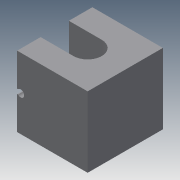
# Autodesk Inventor part: uchyty_robot
Saved by Autodesk Inventor 2013 (Build 170138000, 138)
## iProperties
Created: 2013-05-14
Part Number: uchyty_robot
Material: Generic
Document SubType Name: Modeling
Designer: idle-rug
Density: 1 g/cm^3
Author: idle-rug
Autodesk Inventor part; units mm, degrees
ref_plane "YZ Plane" through (0, 0, 0) normal (1, 0, 0) x (0, 1, 0)
ref_plane "XZ Plane" through (0, 0, 0) normal (0, 1, 0) x (-1, 0, 0)
ref_plane "XY Plane" through (0, 0, 0) normal (0, 0, 1) x (1, 0, 0)
sketch "Sketch1" plane through (0, 0, 0) normal (0, 1, 0) x (-1, 0, 0)
  line L0 (15, 10) -> (-15, 10)
  line L1 (-15, 10) -> (-15, -10)
  line L2 (-15, -10) -> (15, -10)
  line L3 (15, -10) -> (15, 10)
  line L4 (15, 10) -> (-15, -10) construction
  line L5 (-15, 10) -> (15, -10) construction
  point P0 (0, 0)
  dimension "d0" = 30
  dimension "d1" = 20
  constraints: 12 end point, 2 midpoint, 2 parallel, 1 horizontal, 1 perpendicular
  measures "d0" distance of L2.end L1.end
  measures "d1" distance of L1.end L0.end
extrude "Extrusion1" add sketch "Sketch1" along normal blind 10
sketch "Sketch2" plane through (0, 10, 0) normal (0, 1, 0) x (1, 0, 0)
  line L0 (-15, 10) -> (-15, -10) projected
  line L1 (-15, 0) -> (-12, 0)
  circle A0 centre (-13.5, 0) radius 1.5
  point P0 (0, 0)
  dimension "d4" = 3
  constraints: 2 end point, 2 midpoint, 1 centre point, 1 perpendicular, 1 tangent
  measures "d4" distance of L1.start L1.end
extrude "Extrusion2" cut sketch "Sketch2" against normal blind 10
sketch "Sketch3" plane through (0, 10, 0) normal (0, 1, 0) x (1, 0, 0)
  line L0 (-15, 10) -> (-15, 0) projected
  circle A0 centre (-13.5, 0) radius 1.5 projected
  line L1 (-15, 0) -> (-15, -10) projected
  line L2 (-15, 0) -> (-15, 1)
  line L3 (-15, 1) -> (-14.618, 1)
  line L4 (-15, 0) -> (-15, -1)
  line L5 (-15, -1) -> (-14.618, -1)
  point P0 (0, 0)
  dimension "d7" = 1
  dimension "d8" = 1
  constraints: 8 end point, 2 perpendicular, 2 point on circle, 2 point on line
  measures "d7" distance of L0.end L2.end
  measures "d8" distance of L0.end L4.end
extrude "Extrusion3" add sketch "Sketch3" against normal blind 10 contours L3 A0 L0 | A0 L5 L1
sketch "Sketch4" plane through (0, 10, 0) normal (0, 1, 0) x (1, 0, 0)
  circle A0 centre (-13.5, 0) radius 1.5 projected
  line L0 (-15.382, 1) -> (-14.618, 1)
  line L1 (-14.618, 1) -> (-14.618, -1)
  line L2 (-14.618, -1) -> (-15.382, -1)
  line L3 (-15.382, -1) -> (-15.382, 1)
  line L4 (-15.382, 1) -> (-14.618, -1) construction
  line L5 (-14.618, 1) -> (-15.382, -1) construction
  point P0 (0, 0)
  dimension "d11" = 2
  constraints: 12 end point, 2 parallel, 1 horizontal, 1 perpendicular, 2 other
  measures "d11" distance of L0.end L1.end
extrude "Extrusion4" cut sketch "Sketch4" against normal blind 10 contours L1 A0 | A0 L2 L3 L0 picked at (-14.7453, 0)
sketch "Sketch5" plane through (0, 0, 0) normal (0, -1, 0) x (1, 0, 0)
  line L0 (-15, 10) -> (15, 10) projected
  line L1 (15, -10) -> (5, -10)
  line L2 (5, -10) -> (5, 10)
  line L3 (5, 10) -> (15, 10)
  line L4 (15, 10) -> (15, -10)
  point P0 (0, 0)
  dimension "d14" = 10
  constraints: 8 end point, 2 parallel, 1 horizontal, 1 perpendicular, 1 point on line
  measures "d14" distance of L2.end L3.end
extrude "Extrusion5" add sketch "Sketch5" along normal blind 12
sketch "Sketch6" plane through (15, 10, 10) normal (1, 0, 0) x (0, 0, -1)
  line L0 (0, -22) -> (20, -22)
  line L1 (20, -22) -> (20, -32)
  line L2 (20, -32) -> (0, -32)
  line L3 (0, -32) -> (0, -22)
  point P0 (10, -10)
  dimension "d17" = 10
  constraints: 8 end point, 2 parallel, 1 horizontal, 1 perpendicular
  measures "d17" distance of L0.end L1.end
extrude "Extrusion6" add sketch "Sketch6" against normal blind 30
sketch "Sketch7" plane through (15, -22, -10) normal (0, -1, 0) x (1, 0, 0)
  circle A0 centre (-28.5, 10) radius 1.5
  point P0 (-15, 10)
  constraints: 1 centre point
extrude "Extrusion7" cut sketch "Sketch7" against normal blind 10
sketch "Sketch8" plane through (15, -22, -10) normal (0, -1, 0) x (1, 0, 0)
  circle A0 centre (-28.5, 10) radius 1.5 projected
  line L0 (-30.382, 11) -> (-29.618, 11)
  line L1 (-29.618, 11) -> (-29.618, 9)
  line L2 (-29.618, 9) -> (-30.382, 9)
  line L3 (-30.382, 9) -> (-30.382, 11)
  line L4 (-30.382, 11) -> (-29.618, 9) construction
  line L5 (-29.618, 11) -> (-30.382, 9) construction
  point P0 (-15, 10)
  dimension "d23" = 2
  constraints: 12 end point, 2 parallel, 1 horizontal, 1 perpendicular, 2 other
  measures "d23" distance of L0.end L1.end
extrude "Extrusion8" cut sketch "Sketch8" against normal blind 10 contours L1 A0 | A0 L2 L3 L0 picked at (-29.7453, 10)
fillet "Fillet1" radius 6 2 edges at (5, 0, 0) (5, -12, 0)
sketch "Sketch9" plane through (15, 10, -10) normal (0, 0, -1) x (-1, 0, 0)
  line L0 (16, -10) -> (30, -10) projected
  line L1 (30, -10) -> (30, 0) projected
  line L2 (0, 0) -> (30, 0) projected
  line L3 (0, -32) -> (0, 0) projected
  line L4 (0, -32) -> (30, -32) projected
  line L5 (30, -22) -> (30, -32) projected
  line L6 (16, -22) -> (30, -22) projected
  arc A0 (16, -10) -> (16, -22) centre (16, -16) ccw projected
  point P0 (15, -10)
extrude "Extrusion9" add sketch "Sketch9" along normal blind 5
sketch "Sketch10" plane through (-15, 10, 10) normal (0, 0, 1) x (1, 0, 0)
  line L0 (0, -10) -> (14, -10) projected
  arc A0 (14, -22) -> (14, -10) centre (14, -16) ccw projected
  line L1 (14, -22) -> (0, -22) projected
  line L2 (0, -32) -> (0, -22) projected
  line L3 (30, -32) -> (0, -32) projected
  line L4 (30, -32) -> (30, 0) projected
  line L5 (0, 0) -> (30, 0) projected
  line L6 (0, -10) -> (0, 0) projected
  point P0 (15, -10)
extrude "Extrusion10" add sketch "Sketch10" along normal blind 5
sketch "Sketch12" plane through (-15, 10, 10) normal (-1, 0, 0) x (0, 0, 1)
  circle A0 centre (-2, -27) radius 1.5
  point P0 (-10, -10)
  dimension "d31" = 3
  constraints: 1 centre point
  measures "d31" diameter of A0
sketch "Sketch13" plane through (-15, 10, 10) normal (-1, 0, 0) x (0, 0, 1)
  circle A0 centre (-18, -27) radius 1.5
  point P0 (-10, -10)
  dimension "d32" = 3
  constraints: 1 centre point
  measures "d32" diameter of A0
sketch "Sketch14" plane through (-15, 0, -1) normal (-1, 0, 0) x (0, 0, 1)
  circle A0 centre (-7, 5) radius 1.5
  point P0 (1, 0)
  dimension "d33" = 3
  constraints: 1 centre point
  measures "d33" diameter of A0
sketch "Sketch15" plane through (-15, 0, 1) normal (-1, 0, 0) x (0, 0, 1)
  circle A0 centre (7, 5) radius 1.5
  point P0 (-1, 0)
  dimension "d34" = 3
  constraints: 1 centre point
  measures "d34" diameter of A0
extrude "Extrusion11" cut sketch "Sketch14" against normal blind 5
extrude "Extrusion12" cut sketch "Sketch15" against normal blind 5
extrude "Extrusion13" cut sketch "Sketch13" against normal blind 5
extrude "Extrusion14" cut sketch "Sketch12" against normal blind 5
sketch "Sketch17" plane through (-15, 10, 10) normal (-1, 0, 0) x (0, 0, 1)
  circle A0 centre (-2, -27) radius 1.5 projected
  point P0 (-10, -10)
sketch "Sketch18" plane through (-15, 10, 10) normal (-1, 0, 0) x (0, 0, 1)
  circle A0 centre (-18, -27) radius 1.5 projected
  point P0 (-10, -10)
sketch "Sketch19" plane through (-15, 0, -1) normal (-1, 0, 0) x (0, 0, 1)
  circle A0 centre (-7, 5) radius 1.5 projected
  point P0 (1, 0)
sketch "Sketch20" plane through (-15, 0, 1) normal (-1, 0, 0) x (0, 0, 1)
  circle A0 centre (7, 5) radius 1.5 projected
  point P0 (-1, 0)
extrude "Extrusion15" add sketch "Sketch18" against normal blind 5
extrude "Extrusion16" add sketch "Sketch17" against normal blind 5
extrude "Extrusion17" add sketch "Sketch19" against normal blind 5
extrude "Extrusion18" add sketch "Sketch20" against normal blind 5
sketch "Sketch21" plane through (-15, 10, 10) normal (-1, 0, 0) x (0, 0, 1)
  line L0 (-9, -22) -> (5, -22) projected
  line L1 (-2, -22) -> (-2, -26)
  circle A0 centre (-2, -26) radius 1.5
  point P0 (-10, -10)
  dimension "d51" = 4
  dimension "d52" = 3
  constraints: 2 end point, 1 centre point, 1 coincident, 1 midpoint
  measures "d51" distance of L1.start L1.end
  measures "d52" diameter of A0
sketch "Sketch22" plane through (-15, 10, 10) normal (-1, 0, 0) x (0, 0, 1)
  line L0 (-11, -22) -> (-25, -22) projected
  line L1 (-18, -22) -> (-18, -26)
  circle A0 centre (-18, -26) radius 1.5
  point P0 (-10, -10)
  dimension "d53" = 4
  dimension "d54" = 3
  constraints: 2 end point, 1 centre point, 1 coincident, 1 midpoint
  measures "d53" distance of L1.start L1.end
  measures "d54" diameter of A0
sketch "Sketch23" plane through (-15, 0, -1) normal (-1, 0, 0) x (0, 0, 1)
  line L0 (0, 0) -> (-14, 0) projected
  line L1 (-7, 0) -> (-7, 4)
  circle A0 centre (-7, 4) radius 1.5
  point P0 (1, 0)
  dimension "d55" = 4
  dimension "d56" = 3
  constraints: 2 end point, 1 centre point, 1 coincident, 1 midpoint, 1 perpendicular
  measures "d55" distance of L1.start L1.end
  measures "d56" diameter of A0
sketch "Sketch24" plane through (-15, 0, 1) normal (-1, 0, 0) x (0, 0, 1)
  line L0 (0, 0) -> (14, 0) projected
  line L1 (7, 0) -> (7, 4)
  circle A0 centre (7, 4) radius 1.5
  point P0 (-1, 0)
  dimension "d57" = 4
  dimension "d58" = 3
  constraints: 2 end point, 1 centre point, 1 coincident, 1 midpoint
  measures "d57" distance of L1.start L1.end
  measures "d58" diameter of A0
hole "Hole1" at (-15, -16, -8) at (-15, -16, -8) direction (1, 0, 0) diameter 2.459 depth 8 tip angle 118 thread size "M3x0.5" class "6H" standard "ISO Metric profile"
hole "Hole2" at (-15, -16, 8) direction (1, 0, 0) diameter 2.459 depth 8 tip angle 118 thread size "M3x0.5" class "6H" standard "ISO Metric profile"
hole "Hole3" at (-15, 4, 8) direction (1, 0, 0) diameter 2.459 depth 8 tip angle 118 thread size "M3x0.5" class "6H" standard "ISO Metric profile"
hole "Hole4" at (-15, 4, -8) direction (1, 0, 0) diameter 2.459 depth 8 tip angle 118 thread size "M3x0.5" class "6H" standard "ISO Metric profile"
equation "\"d60\" = d54"
equation "\"d67\" = d54"
equation "\"d74\" = d54"
equation "\"d81\" = d54"
body "Solid1"
